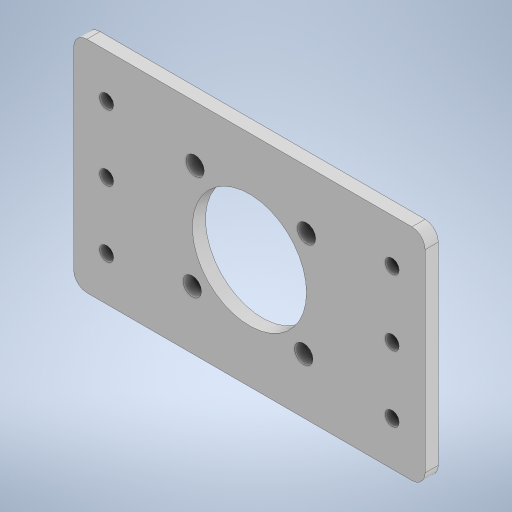
# Autodesk Inventor part: 射出_モーター固定1
Saved by Autodesk Inventor 2023 (Build 270158000, 158)
## iProperties
Created: 2022-04-19
Part Number: 射出_モーター固定1
Material: 一般
Document SubType Name: Modeling
Designer: yuta
Density: 1 g/cm^3
Appearance: 既定
Author: yuta
Autodesk Inventor part; units mm, degrees
ref_plane "YZ Plane" through (0, 0, 0) normal (1, 0, 0) x (0, 1, 0)
ref_plane "XZ Plane" through (0, 0, 0) normal (0, 1, 0) x (-1, 0, 0)
ref_plane "XY Plane" through (0, 0, 0) normal (0, 0, 1) x (1, 0, 0)
sketch "スケッチ1" plane through (0, 0, 0) normal (0, 0, 1) x (1, 0, 0)
  line L0 (0, 0) -> (80, 0)
  line L1 (80, 0) -> (80, 50)
  line L2 (80, 50) -> (0, 50)
  line L3 (0, 50) -> (0, 0)
  dimension "d0" = 80
  dimension "d1" = 50
  constraints: 8 end point, 2 parallel, 1 horizontal, 1 perpendicular
  measures "d0" distance of L2.end L1.end
  measures "d1" distance of L1.end L0.end
extrude "押し出し1" add sketch "スケッチ1" along normal blind 3
sketch "スケッチ2" plane through (0, 0, 3) normal (0, 0, 1) x (1, 0, 0)
  circle A0 centre (40, 25) radius 13
  line L0 (80, 50) -> (0, 50) projected
  line L1 (0, 50) -> (0, 0) projected
  dimension "d4" = 26
  dimension "d5" = 25
  dimension "d6" = 40
  constraints: 1 centre point
  measures "d4" diameter of A0
  measures "d5" distance from line of L0 A0.centre
  measures "d6" distance from line of L1 A0.centre
extrude "押し出し2" cut sketch "スケッチ2" against normal blind 3
sketch "スケッチ3" plane through (0, 0, 3) normal (0, 0, 1) x (1, 0, 0)
  circle A0 centre (40, 25) radius 13 projected
  circle A1 centre (40, 25) radius 17.5 construction
  line L0 (40, 25) -> (57.5, 25)
  line L1 (40, 25) -> (53, 36.7154) construction
  line L2 (53, 36.7154) -> (19.5714, 6.5901) construction
  line L3 (40, 25) -> (52.3744, 12.6256)
  line L4 (40, 25) -> (57.5, 25) construction
  line L5 (52.3744, 12.6256) -> (27.6256, 37.3744) construction
  circle A2 centre (53, 36.7154) radius 2.1
  circle A3 centre (27.6256, 37.3744) radius 2.1
  circle A4 centre (27, 13.2846) radius 2.1
  circle A5 centre (52.3744, 12.6256) radius 2.1
  point P0 (0, 0)
  dimension "d9" = 35
  dimension "d10" = 17.5
  dimension "d11" = 45
  dimension "d12" = 45
  dimension "d13" = 4.2
  dimension "d14" = 4.2
  dimension "d15" = 4.2
  dimension "d16" = 4.2
  constraints: 12 end point, 5 centre point, 4 coincident, 4 point on circle, 3 point on line, 2 horizontal, 1 equal length
  measures "d9" diameter of A1
  measures "d10" distance of L0.start L1.end
  measures "d11" distance of L1.end L2.end
  measures "d12" angle of L3 L4
  measures "d13" diameter of A2
  measures "d14" diameter of A3
  measures "d15" diameter of A4
  measures "d16" diameter of A5
hole "穴1" at (27.6256, 37.3744, 3) at (53, 36.7154, 3) at (27, 13.2846, 3) at (52.3744, 12.6256, 3) direction (0, 0, -1) diameter 4.2 end through all
sketch "スケッチ4" plane through (0, 0, 3) normal (0, 0, 1) x (1, 0, 0)
  line L0 (80, 50) -> (0, 50) projected
  line L1 (15, 50) -> (15, 0) construction
  line L2 (0, 0) -> (80, 0) projected
  line L3 (65, 50) -> (65, 0) construction
  line L4 (0, 50) -> (0, 0) projected
  line L5 (80, 0) -> (80, 50) projected
  circle A0 centre (7.5, 40) radius 1.6
  circle A1 centre (7.5, 25) radius 1.6
  circle A2 centre (7.5, 10) radius 1.6
  circle A3 centre (72.5, 40) radius 1.6
  circle A4 centre (72.5, 25) radius 1.6
  circle A5 centre (72.5, 10) radius 1.6
  point P0 (40, 0)
  dimension "d24" = 15
  dimension "d25" = 15
  dimension "d26" = 3.2
  dimension "d27" = 7.5
  dimension "d28" = 10
  dimension "d29" = 3.2
  dimension "d30" = 3.2
  dimension "d31" = 25
  dimension "d32" = 10
  dimension "d33" = 7.5
  dimension "d34" = 7.5
  constraints: 6 centre point, 4 end point, 4 point on line, 3 equal radius, 3 horizontal alignment, 1 midpoint, 1 perpendicular, 1 vertical, 2 other
  measures "d24" distance between parallel lines of L4 L1
  measures "d25" distance between parallel lines of L5 L3
  measures "d26" diameter of A0
  measures "d27" distance from line of L4 A0.centre
  measures "d28" distance from line of L0 A0.centre
  measures "d29" diameter of A1
  measures "d30" diameter of A2
  measures "d31" distance from line of L0 A1.centre
  measures "d32" distance from line of L2 A2.centre
  measures "d33" distance from line of L4 A2.centre
  measures "d34" distance from line of L4 A1.centre
hole "穴2" at (7.5, 40, 3) at (7.5, 25, 3) at (7.5, 10, 3) at (72.5, 40, 3) at (72.5, 25, 3) at (72.5, 10, 3) direction (0, 0, -1) diameter 3.2 end through all
fillet "フィレット1" radius 3 4 edges at (0, 50, 1.5) (80, 50, 1.5) (80, 0, 1.5) (0, 0, 1.5)
